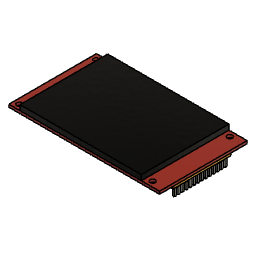
显示屏 v2 (Autodesk Fusion 360 design; units mm, degrees)
Autodesk Fusion 360 part; units mm, degrees
sketch "草图1" plane through (0, 0, 0) normal (0, 0, 1) x (1, 0, 0)
  line L0 (0, 0) -> (6.4, 0)
  line L1 (6.4, 0) -> (6.4, 50)
  line L2 (6.4, 50) -> (0, 50)
  line L3 (0, 50) -> (0, 0)
  line L4 (6.4, 50) -> (75.6, 50)
  line L5 (75.6, 50) -> (75.6, 0)
  line L6 (75.6, 0) -> (6.4, 0)
  line L7 (6.4, 0) -> (6.4, 50)
  line L8 (75.6, 50) -> (86, 50)
  line L9 (86, 50) -> (86, 0)
  line L10 (86, 0) -> (75.6, 0)
  line L11 (75.6, 0) -> (75.6, 50)
  line L12 (-10, 25) -> (111.3719, 25)
  circle A0 centre (3, 3) radius 1.5
  circle A1 centre (3, 47) radius 1.5
  circle A2 centre (79.08, 47) radius 1.5
  circle A3 centre (79.08, 3) radius 1.5
  dimension "d1" = 50
  dimension "d2" = 6.4
  dimension "d3" = 69.2
  dimension "d4" = 10.4
  dimension "d5" = 3
  dimension "d6" = 3
  dimension "d7" = 3
  dimension "d8" = 50
  dimension "d9" = 3
  dimension "d10" = 3
  dimension "d11" = 6.92
  constraint horizontal L0
  constraint vertical L1
  constraint horizontal L2
  constraint vertical L3
  constraint coincident L0.start L3.end
  constraint horizontal L4
  constraint vertical L5
  constraint horizontal L6
  constraint vertical L7
  constraint horizontal L8
  constraint vertical L9
  constraint horizontal L10
  constraint vertical L11
  constraint horizontal L12
  constraint symmetric L12 A0 A1
  constraint symmetric L4 L6 L12
  constraint symmetric L12 A2 A3
  measures "d1" distance of L0.start L2.end
  measures "d2" distance of L1.end L2.end
  measures "d3" distance of L1.end L4.end
  measures "d4" distance of L4.end L8.end
  measures "d5" diameter of A0
  measures "d6" distance of L3 A0.centre
  measures "d7" distance of L0 A0.centre
  measures "d8" distance of L4.end L5.end
  measures "d9" diameter of A2
  measures "d10" distance of L8 A2.centre
  measures "d11" distance of L9 A2.centre
extrude "拉伸1" add sketch "草图1" along normal blind 1.5 makes body 1
sketch "草图2" plane through (0, 0, 1.5) normal (0, 0, 1) x (-1, 0, 0)
  circle A0 centre (-3, -47) radius 1.5
  circle A1 centre (-79.08, -47) radius 1.5
  circle A2 centre (-3, -3) radius 1.5
  circle A3 centre (-79.08, -3) radius 1.5
  line L0 (-86, -50) -> (0, -50)
  line L1 (0, -50) -> (0, 0)
  line L2 (0, 0) -> (-86, 0)
  line L3 (-86, 0) -> (-86, -50)
  line L4 (-6.4, -50) -> (-75.6, -50)
  line L5 (-75.6, -50) -> (-75.6, 0)
  line L6 (-75.6, 0) -> (-6.4, 0)
  line L7 (-6.4, 0) -> (-6.4, -50)
  dimension "d14" = 69.2
  dimension "d15" = 6.4
  constraint horizontal L4
  constraint vertical L5
  constraint horizontal L6
  constraint vertical L7
  constraint coincident L2 L5.end
  constraint coincident L0 L4.start
  measures "d14" distance of L4.start L4.end
  measures "d15" distance of L1 L7
extrude "拉伸2" add sketch "草图2" along normal blind 3 separate body contours L0 L2 L4 L5 L6 L7 makes body 2
sketch "草图3" plane through (0, 0, 0) normal (0, 0, -1) x (1, 0, 0)
  circle A0 centre (3, -47) radius 1.5
  circle A1 centre (79.08, -47) radius 1.5
  circle A2 centre (3, -3) radius 1.5
  circle A3 centre (79.08, -3) radius 1.5
  line L0 (0, -50) -> (86, -50)
  line L1 (86, -50) -> (86, 0)
  line L2 (86, 0) -> (0, 0)
  line L3 (0, 0) -> (0, -50)
  line L4 (82.75, -8.49) -> (85.25, -8.49)
  line L5 (85.25, -8.49) -> (85.25, -41.51)
  line L6 (85.25, -41.51) -> (82.75, -41.51)
  line L7 (82.75, -41.51) -> (82.75, -8.49)
  dimension "d18" = 8.49
  dimension "d19" = 8.49
  dimension "d20" = 2.5
  dimension "d21" = 0.75
  constraint horizontal L4
  constraint vertical L5
  constraint horizontal L6
  constraint vertical L7
  measures "d18" distance of L2 L4
  measures "d19" distance of L0 L6
  measures "d20" distance of L4.start L4.end
  measures "d21" distance of L1 L5
extrude "拉伸3" add sketch "草图3" along normal blind 2 separate body contours L4 L5 L6 L7 makes body 3
sketch "草图4" plane through (0, 0, -2) normal (0, 0, -1) x (1, 0, 0)
  line L0 (82.75, -41.51) -> (85.25, -41.51)
  line L1 (85.25, -41.51) -> (85.25, -8.49)
  line L2 (85.25, -8.49) -> (82.75, -8.49)
  line L3 (82.75, -8.49) -> (82.75, -41.51)
  line L4 (84.5, -11) -> (83.5404, -11)
  line L5 (83.5404, -11) -> (83.5404, -9.9)
  line L6 (83.5404, -9.9) -> (84.5, -9.9)
  line L7 (84.5, -9.9) -> (84.5, -11)
  line L8 (84.5, -11) -> (83.5404, -9.9) construction
  line L9 (83.5404, -11) -> (84.5, -9.9) construction
  line L10 (83.5404, -13.2308) -> (83.5404, -12.1308)
  line L11 (84.5, -13.2308) -> (83.5404, -13.2308)
  line L12 (83.5404, -12.1308) -> (84.5, -12.1308)
  line L13 (84.5, -12.1308) -> (84.5, -13.2308)
  line L14 (83.5404, -15.4615) -> (83.5404, -14.3615)
  line L15 (84.5, -15.4615) -> (83.5404, -15.4615)
  line L16 (83.5404, -14.3615) -> (84.5, -14.3615)
  line L17 (84.5, -14.3615) -> (84.5, -15.4615)
  line L18 (83.5404, -17.6923) -> (83.5404, -16.5923)
  line L19 (84.5, -17.6923) -> (83.5404, -17.6923)
  line L20 (83.5404, -16.5923) -> (84.5, -16.5923)
  line L21 (84.5, -16.5923) -> (84.5, -17.6923)
  line L22 (83.5404, -19.9231) -> (83.5404, -18.8231)
  line L23 (84.5, -19.9231) -> (83.5404, -19.9231)
  line L24 (83.5404, -18.8231) -> (84.5, -18.8231)
  line L25 (84.5, -18.8231) -> (84.5, -19.9231)
  line L26 (83.5404, -22.1538) -> (83.5404, -21.0538)
  line L27 (84.5, -22.1538) -> (83.5404, -22.1538)
  line L28 (83.5404, -21.0538) -> (84.5, -21.0538)
  line L29 (84.5, -21.0538) -> (84.5, -22.1538)
  line L30 (83.5404, -24.3846) -> (83.5404, -23.2846)
  line L31 (84.5, -24.3846) -> (83.5404, -24.3846)
  line L32 (83.5404, -23.2846) -> (84.5, -23.2846)
  line L33 (84.5, -23.2846) -> (84.5, -24.3846)
  line L34 (83.5404, -26.6154) -> (83.5404, -25.5154)
  line L35 (84.5, -26.6154) -> (83.5404, -26.6154)
  line L36 (83.5404, -25.5154) -> (84.5, -25.5154)
  line L37 (84.5, -25.5154) -> (84.5, -26.6154)
  line L38 (83.5404, -28.8462) -> (83.5404, -27.7462)
  line L39 (84.5, -28.8462) -> (83.5404, -28.8462)
  line L40 (83.5404, -27.7462) -> (84.5, -27.7462)
  line L41 (84.5, -27.7462) -> (84.5, -28.8462)
  line L42 (83.5404, -31.0769) -> (83.5404, -29.9769)
  line L43 (84.5, -31.0769) -> (83.5404, -31.0769)
  line L44 (83.5404, -29.9769) -> (84.5, -29.9769)
  line L45 (84.5, -29.9769) -> (84.5, -31.0769)
  line L46 (83.5404, -33.3077) -> (83.5404, -32.2077)
  line L47 (84.5, -33.3077) -> (83.5404, -33.3077)
  line L48 (83.5404, -32.2077) -> (84.5, -32.2077)
  line L49 (84.5, -32.2077) -> (84.5, -33.3077)
  line L50 (83.5404, -35.5385) -> (83.5404, -34.4385)
  line L51 (84.5, -35.5385) -> (83.5404, -35.5385)
  line L52 (83.5404, -34.4385) -> (84.5, -34.4385)
  line L53 (84.5, -34.4385) -> (84.5, -35.5385)
  line L54 (83.5404, -37.7692) -> (83.5404, -36.6692)
  line L55 (84.5, -37.7692) -> (83.5404, -37.7692)
  line L56 (83.5404, -36.6692) -> (84.5, -36.6692)
  line L57 (84.5, -36.6692) -> (84.5, -37.7692)
  line L58 (83.5404, -40) -> (83.5404, -38.9)
  line L59 (84.5, -40) -> (83.5404, -40)
  line L60 (83.5404, -38.9) -> (84.5, -38.9)
  line L61 (84.5, -38.9) -> (84.5, -40)
  point P0 (84.0202, -10.45)
  dimension "d26" = 0
  dimension "d27" = -29
  constraint horizontal L4
  constraint perpendicular L4 L5
  constraint parallel L4 L6
  constraint parallel L5 L7
  constraint coincident L8 P0
  constraint coincident L9 P0
extrude "拉伸4" add sketch "草图4" along normal blind 5 separate body contours L4 L5 L6 L7 | L10 L11 L12 L13 | L14 L15 L16 L17 | L18 L19 L20 L21 | L22 L23 L24 L25 | L26 L27 L28 L29 | L30 L31 L32 L33 | L34 L35 L36 L37 | L38 L39 L40 L41 | L42 L43 L44 L45 | L46 L47 L48 L49 | L50 L51 L52 L53 | L54 L55 L56 L57 | L58 L59 L60 L61 makes body 4 at (83.5404, 30.7103, -3.6667) makes body 5 at (83.5404, 21.7872, -3.6667) makes body 6 at (83.5404, 12.8641, -3.6667) makes body 7 at (83.5404, 39.6333, -3.6667) makes body 8 at (83.5404, 15.0949, -3.6667) makes body 9 at (83.5404, 24.0179, -3.6667) makes body 10 at (83.5404, 32.941, -3.6667) makes body 11 at (83.5404, 28.4795, -3.6667) makes body 12 at (83.5404, 19.5564, -3.6667) makes body 13 at (83.5404, 10.6333, -3.6667) makes body 14 at (83.5404, 37.4026, -3.6667) makes body 15 at (83.5404, 17.3256, -3.6667) makes body 16 at (83.5404, 26.2487, -3.6667) makes body 17 at (84.5, 34.8051, -3.6667)
copy_body "实体->零部件1" bodies 1 removing the originals makes body 18 in component "Component'"
copy_body "实体->零部件2" bodies 2 removing the originals makes body 19 in component "Component''"
copy_body "实体->零部件3" bodies 3 removing the originals makes body 20 in component "Component'''"
copy_body "实体->零部件4" bodies 4 removing the originals makes body 21 in component "Component''''"
copy_body "实体->零部件5" bodies 5 removing the originals makes body 22 in component "Component'''''"
copy_body "实体->零部件6" bodies 6 removing the originals makes body 23 in component "Component''''''"
copy_body "实体->零部件7" bodies 7 removing the originals makes body 24 in component "Component'''''''"
copy_body "实体->零部件8" bodies 8 removing the originals makes body 25 in component "Component''''''''"
copy_body "实体->零部件9" bodies 9 removing the originals makes body 26 in component "Component'''''''''"
copy_body "实体->零部件10" bodies 10 removing the originals makes body 27 in component "Component''''''''''"
copy_body "实体->零部件11" bodies 11 removing the originals makes body 28 in component "Component'''''''''''"
copy_body "实体->零部件12" bodies 12 removing the originals makes body 29 in component "Component''''''''''''"
copy_body "实体->零部件13" bodies 13 removing the originals makes body 30 in component "Component'''''''''''''"
copy_body "实体->零部件14" bodies 14 removing the originals makes body 31 in component "Component''''''''''''''"
copy_body "实体->零部件15" bodies 15 removing the originals makes body 32 in component "Component'''''''''''''''"
copy_body "实体->零部件16" bodies 16 removing the originals makes body 33 in component "Component''''''''''''''''"
copy_body "实体->零部件17" bodies 17 removing the originals makes body 34 in component "Component'''''''''''''''''"
component "Component'" placed x (1, 0, 0) y (0, 1, 0) z (0, 0, 1) at (0, 0, 0)
component "Component''" placed x (1, 0, 0) y (0, 1, 0) z (0, 0, 1) at (0, 0, 0)
component "Component'''" placed x (1, 0, 0) y (0, 1, 0) z (0, 0, 1) at (0, 0, 0)
component "Component''''" placed x (1, 0, 0) y (0, 1, 0) z (0, 0, 1) at (0, 0, 0)
component "Component'''''" placed x (1, 0, 0) y (0, 1, 0) z (0, 0, 1) at (0, 0, 0)
component "Component''''''" placed x (1, 0, 0) y (0, 1, 0) z (0, 0, 1) at (0, 0, 0)
component "Component'''''''" placed x (1, 0, 0) y (0, 1, 0) z (0, 0, 1) at (0, 0, 0)
component "Component''''''''" placed x (1, 0, 0) y (0, 1, 0) z (0, 0, 1) at (0, 0, 0)
component "Component'''''''''" placed x (1, 0, 0) y (0, 1, 0) z (0, 0, 1) at (0, 0, 0)
component "Component''''''''''" placed x (1, 0, 0) y (0, 1, 0) z (0, 0, 1) at (0, 0, 0)
component "Component'''''''''''" placed x (1, 0, 0) y (0, 1, 0) z (0, 0, 1) at (0, 0, 0)
component "Component''''''''''''" placed x (1, 0, 0) y (0, 1, 0) z (0, 0, 1) at (0, 0, 0)
component "Component'''''''''''''" placed x (1, 0, 0) y (0, 1, 0) z (0, 0, 1) at (0, 0, 0)
component "Component''''''''''''''" placed x (1, 0, 0) y (0, 1, 0) z (0, 0, 1) at (0, 0, 0)
component "Component'''''''''''''''" placed x (1, 0, 0) y (0, 1, 0) z (0, 0, 1) at (0, 0, 0)
component "Component''''''''''''''''" placed x (1, 0, 0) y (0, 1, 0) z (0, 0, 1) at (0, 0, 0)
component "Component'''''''''''''''''" placed x (1, 0, 0) y (0, 1, 0) z (0, 0, 1) at (0, 0, 0)
